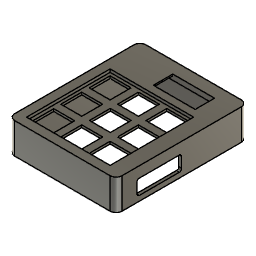
bdn9-top-case (Autodesk Fusion 360 design; units mm, degrees)
Autodesk Fusion 360 part; units mm, degrees
note: some values were not read from the file. Chosen so that the rebuilt part matches the saved one: which face or edge a step refers to; which pieces of a blend or face edit are solid.
sketch "Sketch1" plane through (0, 0, 0) normal (0, 0, 1) x (1, 0, 0)
  line L0 (-8, -80) -> (-22, -80)
  line L1 (-22, -80) -> (-22, -66)
  line L2 (-22, -66) -> (-8, -66)
  line L3 (-8, -66) -> (-8, -80)
  line L4 (-8, -61) -> (-22, -61)
  line L5 (-22, -61) -> (-22, -47)
  line L6 (-22, -47) -> (-8, -47)
  line L7 (-8, -47) -> (-8, -61)
  line L8 (-8, -42) -> (-22, -42)
  line L9 (-22, -42) -> (-22, -28)
  line L10 (-22, -28) -> (-8, -28)
  line L11 (-8, -28) -> (-8, -42)
  line L12 (0, 0) -> (-68, 0)
  line L13 (-68, 0) -> (-68, -88)
  line L14 (-68, -88) -> (0, -88)
  line L15 (0, -88) -> (0, 0)
  line L16 (-27, -28) -> (-41, -28)
  line L17 (-41, -28) -> (-41, -42)
  line L18 (-41, -42) -> (-27, -42)
  line L19 (-27, -42) -> (-27, -28)
  line L20 (-27, -46.8468) -> (-41, -46.8468)
  line L21 (-41, -46.8468) -> (-41, -60.8468)
  line L22 (-41, -60.8468) -> (-27, -60.8468)
  line L23 (-27, -60.8468) -> (-27, -46.8468)
  line L24 (-27, -66) -> (-41, -66)
  line L25 (-41, -66) -> (-41, -80)
  line L26 (-41, -80) -> (-27, -80)
  line L27 (-27, -80) -> (-27, -66)
  line L28 (-46, -28) -> (-60, -28)
  line L29 (-60, -28) -> (-60, -42)
  line L30 (-60, -42) -> (-46, -42)
  line L31 (-46, -42) -> (-46, -28)
  line L32 (-46, -47) -> (-60, -47)
  line L33 (-60, -47) -> (-60, -61)
  line L34 (-60, -61) -> (-46, -61)
  line L35 (-46, -61) -> (-46, -47)
  line L36 (-45.7846, -66) -> (-59.7846, -66)
  line L37 (-59.7846, -66) -> (-59.7846, -80)
  line L38 (-59.7846, -80) -> (-45.7846, -80)
  line L39 (-45.7846, -80) -> (-45.7846, -66)
  line L40 (-5, -8) -> (-44, -8)
  line L41 (-44, -8) -> (-44, -21)
  line L42 (-44, -21) -> (-5, -21)
  line L43 (-5, -21) -> (-5, -8)
  dimension "d15" = 68
  dimension "d16" = 88
  dimension "d29" = 39
  dimension "d30" = 13
  constraint horizontal L0
  constraint vertical L1
  constraint horizontal L2
  constraint vertical L3
  constraint horizontal L4
  constraint vertical L5
  constraint horizontal L6
  constraint vertical L7
  constraint horizontal L8
  constraint vertical L9
  constraint horizontal L10
  constraint vertical L11
  constraint horizontal L12
  constraint vertical L13
  constraint horizontal L14
  constraint vertical L15
  constraint coincident L12.start L15.end
  constraint horizontal L16
  constraint vertical L17
  constraint horizontal L18
  constraint vertical L19
  constraint horizontal L20
  constraint vertical L21
  constraint horizontal L22
  constraint vertical L23
  constraint horizontal L24
  constraint vertical L25
  constraint horizontal L26
  constraint vertical L27
  constraint horizontal L28
  constraint vertical L29
  constraint horizontal L30
  constraint vertical L31
  constraint horizontal L32
  constraint vertical L33
  constraint horizontal L34
  constraint vertical L35
  constraint horizontal L36
  constraint vertical L37
  constraint horizontal L38
  constraint vertical L39
  constraint horizontal L40
  constraint vertical L41
  constraint horizontal L42
  constraint vertical L43
  measures "d15" distance of L12.start L12.end
  measures "d16" distance of L12.start L14.end
  measures "d29" distance of L40.start L40.end
  measures "d30" distance of L40.start L42.end
extrude "Extrude1" add sketch "Sketch1" along normal blind 2
extrude "Extrude2" cut 1 faces at (-57.3333, -12, 2) along direction (0, 0, -1) blind 0.4
extrude "Extrude3" add 1 faces at (0, -58.6667, 0.5333) along direction (1, 0, 0) blind 2
sketch "Sketch2" plane through (0, 0, 1.6) normal (0, 0, 1) x (-1, 0, 0)
  line L0 (27, 66) -> (27, 80)
  line L1 (27, 80) -> (41, 80)
  line L2 (41, 80) -> (41, 66)
  line L3 (41, 66) -> (27, 66)
  line L4 (5, 8) -> (5, 21)
  line L5 (5, 21) -> (44, 21)
  line L6 (44, 21) -> (44, 8)
  line L7 (44, 8) -> (5, 8)
  line L8 (27, 46.8468) -> (27, 60.8468)
  line L9 (27, 60.8468) -> (41, 60.8468)
  line L10 (41, 60.8468) -> (41, 46.8468)
  line L11 (41, 46.8468) -> (27, 46.8468)
  line L12 (22, 47) -> (8, 47)
  line L13 (8, 47) -> (8, 61)
  line L14 (8, 61) -> (22, 61)
  line L15 (22, 61) -> (22, 47)
  line L16 (22, 66) -> (8, 66)
  line L17 (8, 66) -> (8, 80)
  line L18 (8, 80) -> (22, 80)
  line L19 (22, 80) -> (22, 66)
  line L20 (27, 28) -> (27, 42)
  line L21 (27, 42) -> (41, 42)
  line L22 (41, 42) -> (41, 28)
  line L23 (41, 28) -> (27, 28)
  line L24 (22, 28) -> (8, 28)
  line L25 (8, 28) -> (8, 42)
  line L26 (8, 42) -> (22, 42)
  line L27 (22, 42) -> (22, 28)
  line L28 (46, 47) -> (46, 61)
  line L29 (46, 61) -> (60, 61)
  line L30 (60, 61) -> (60, 47)
  line L31 (60, 47) -> (46, 47)
  line L32 (46, 28) -> (46, 42)
  line L33 (46, 42) -> (60, 42)
  line L34 (60, 42) -> (60, 28)
  line L35 (60, 28) -> (46, 28)
  line L36 (45.7846, 66) -> (45.7846, 80)
  line L37 (45.7846, 80) -> (59.7846, 80)
  line L38 (59.7846, 80) -> (59.7846, 66)
  line L39 (59.7846, 66) -> (45.7846, 66)
  line L40 (-2, 0) -> (68, 0)
  line L41 (68, 0) -> (68, 88)
  line L42 (68, 88) -> (-2, 88)
  line L43 (-2, 88) -> (-2, 0)
  line L44 (6, 26) -> (62, 26)
  line L45 (62, 26) -> (62, 82)
  line L46 (62, 82) -> (6, 82)
  line L47 (6, 82) -> (6, 26)
  constraint horizontal L44
  constraint vertical L45
  constraint horizontal L46
  constraint vertical L47
extrude "Extrude4" add sketch "Sketch2" along normal blind 2 contours L40 L41 L42 L43
sketch "Sketch3" plane through (0, 0, 0) normal (0, 0, 1) x (1, 0, 0)
  line L0 (-10, -8) -> (-38, -8)
  line L1 (-38, -8) -> (-38, -21)
  line L2 (-38, -21) -> (-10, -21)
  line L3 (-10, -21) -> (-10, -8)
  line L4 (-38, -8) -> (-44, -8)
  line L5 (-44, -8) -> (-44, -21)
  line L6 (-44, -21) -> (-38, -21)
  line L7 (-38, -21) -> (-38, -8)
  line L8 (-10, -8) -> (-5, -8)
  line L9 (-5, -8) -> (-5, -21)
  line L10 (-5, -21) -> (-10, -21)
  line L11 (-10, -21) -> (-10, -8)
  dimension "d39" = 28
  dimension "d40" = 13
  constraint horizontal L0
  constraint vertical L1
  constraint horizontal L2
  constraint vertical L3
  constraint horizontal L4
  constraint vertical L5
  constraint horizontal L6
  constraint vertical L7
  constraint horizontal L8
  constraint vertical L9
  constraint horizontal L10
  constraint vertical L11
  measures "d39" distance of L0.start L0.end
  measures "d40" distance of L0.start L2.end
move_body "Move1" bodies 1 to x (1, 0, 0) y (0, 1, 0) z (0, 0, 1) at (0, 0, -3)
extrude "Extrude5" add sketch "Sketch3" along normal blind 0.6 contours L3 L8 L9 L10 L11 | L1 L4 L5 L6 L7
extrude "Extrude6" add 2 faces at (-42, -16.6667, 0) (-6.6667, -16.6667, 0) along direction (0, 0, -1) blind 0.4
sketch "Sketch4" plane through (0, 0, 0) normal (0, 0, 1) x (1, 0, 0)
move_body "Move2" bodies 1 to x (1, 0, 0) y (0, 1, 0) z (0, 0, 1) at (0, 0, 0.6)
sketch "Sketch5" plane through (0, 0, 0) normal (0, 0, 1) x (1, 0, 0)
sketch "Sketch6" plane through (0, 0, 0) normal (0, 0, 1) x (1, 0, 0)
sketch "Sketch7" plane through (0, 0, -2.4) normal (0, 0, -1) x (1, 0, 0)
  line L0 (-27, 80) -> (-27, 66)
  line L1 (-27, 66) -> (-41, 66)
  line L2 (-41, 66) -> (-41, 80)
  line L3 (-41, 80) -> (-27, 80)
  line L4 (-5, 21) -> (-5, 8)
  line L5 (-5, 8) -> (-44, 8)
  line L6 (-44, 8) -> (-44, 21)
  line L7 (-44, 21) -> (-5, 21)
  line L8 (-27, 60.8468) -> (-27, 46.8468)
  line L9 (-27, 46.8468) -> (-41, 46.8468)
  line L10 (-41, 46.8468) -> (-41, 60.8468)
  line L11 (-41, 60.8468) -> (-27, 60.8468)
  line L12 (-8, 47) -> (-22, 47)
  line L13 (-22, 47) -> (-22, 61)
  line L14 (-22, 61) -> (-8, 61)
  line L15 (-8, 61) -> (-8, 47)
  line L16 (-8, 66) -> (-22, 66)
  line L17 (-22, 66) -> (-22, 80)
  line L18 (-22, 80) -> (-8, 80)
  line L19 (-8, 80) -> (-8, 66)
  line L20 (-27, 42) -> (-27, 28)
  line L21 (-27, 28) -> (-41, 28)
  line L22 (-41, 28) -> (-41, 42)
  line L23 (-41, 42) -> (-27, 42)
  line L24 (-8, 28) -> (-22, 28)
  line L25 (-22, 28) -> (-22, 42)
  line L26 (-22, 42) -> (-8, 42)
  line L27 (-8, 42) -> (-8, 28)
  line L28 (-46, 61) -> (-46, 47)
  line L29 (-46, 47) -> (-60, 47)
  line L30 (-60, 47) -> (-60, 61)
  line L31 (-60, 61) -> (-46, 61)
  line L32 (-46, 42) -> (-46, 28)
  line L33 (-46, 28) -> (-60, 28)
  line L34 (-60, 28) -> (-60, 42)
  line L35 (-60, 42) -> (-46, 42)
  line L36 (-45.7846, 80) -> (-45.7846, 66)
  line L37 (-45.7846, 66) -> (-59.7846, 66)
  line L38 (-59.7846, 66) -> (-59.7846, 80)
  line L39 (-59.7846, 80) -> (-45.7846, 80)
  line L40 (2, 88) -> (-68, 88)
  line L41 (-68, 88) -> (-68, 0)
  line L42 (-68, 0) -> (2, 0)
  line L43 (2, 0) -> (2, 88)
sketch "Sketch8" plane through (0, 0, 0) normal (0, 0, 1) x (1, 0, 0)
sketch "Sketch9" plane through (0, 0, -2.4) normal (0, 0, -1) x (1, 0, 0)
  line L0 (-2, 84) -> (-64, 84)
  line L1 (-64, 84) -> (-64, 4)
  line L2 (-64, 4) -> (-2, 4)
  line L3 (-2, 4) -> (-2, 84)
  constraint horizontal L0
  constraint vertical L1
  constraint horizontal L2
  constraint vertical L3
extrude "Extrude7" add sketch "Sketch7" along normal blind 17
extrude "Extrude8" cut sketch "Sketch9" along normal blind 17
sketch "Sketch10" plane through (2, 0, 0) normal (1, 0, 0) x (0, 1, 0)
  line L0 (-88, 1.2) -> (-88, -19.4)
  line L1 (-88, -19.4) -> (0, -19.4)
  line L2 (0, -19.4) -> (0, 1.2)
  line L3 (0, 1.2) -> (-88, 1.2)
sketch "Sketch11" plane through (2, 0, 0) normal (1, 0, 0) x (0, 1, 0)
  line L0 (-68, -16) -> (-38, -16)
  line L1 (-38, -16) -> (-38, -6)
  line L2 (-38, -6) -> (-68, -6)
  line L3 (-68, -6) -> (-68, -16)
  dimension "d49" = 30
  dimension "d50" = 10
  constraint horizontal L0
  constraint vertical L1
  constraint horizontal L2
  constraint vertical L3
  measures "d49" distance of L0.start L0.end
  measures "d50" distance of L0.start L2.end
extrude "Extrude9" cut sketch "Sketch11" against normal blind 4
fillet "Fillet1" radius 1.5 1 edges at (0, -68, -6)
fillet "Fillet2" radius 1.5 1 edges at (0, -38, -6)
fillet "Fillet3" radius 1.5 1 edges at (0, -68, -16)
fillet "Fillet4" radius 1.5 1 edges at (0, -38, -16)
fillet "Fillet5" radius 4 1 edges at (2, -88, -9.1)
fillet "Fillet6" radius 4 1 edges at (2, 0, -9.1)
fillet "Fillet7" radius 4 1 edges at (-68, 0, -9.1)
fillet "Fillet8" radius 4 1 edges at (-68, -88, -9.1)
sketch "Sketch12" plane through (0, 0, 0) normal (0, 0, 1) x (1, 0, 0)
  line L0 (-2, -4, -19.4) -> (-11, -4, -19.4)
  line L1 (-11, -4, -19.4) -> (-11, -13, -19.4)
  line L2 (-11, -13, -19.4) -> (-2, -13, -19.4)
  line L3 (-2, -13, -19.4) -> (-2, -4, -19.4)
  dimension "d61" = 9
  dimension "d62" = 9
sketch "Sketch13" plane through (0, 0, -19.4) normal (0, 0, 1) x (1, 0, 0)
  line L0 (-64, -4) -> (-55, -4)
  line L1 (-55, -4) -> (-55, -13)
  line L2 (-55, -13) -> (-64, -13)
  line L3 (-64, -13) -> (-64, -4)
  line L4 (-64, -84) -> (-55, -84)
  line L5 (-55, -84) -> (-55, -75)
  line L6 (-55, -75) -> (-64, -75)
  line L7 (-64, -75) -> (-64, -84)
  line L8 (-2, -84) -> (-11, -84)
  line L9 (-11, -84) -> (-11, -75)
  line L10 (-11, -75) -> (-2, -75)
  line L11 (-2, -75) -> (-2, -84)
  point P0 (-64, -4)
  point P1 (-64, -84)
  point P2 (-2, -84)
  dimension "d63" = 9
  dimension "d64" = 9
  dimension "d65" = 9
  dimension "d66" = 9
  dimension "d67" = 9
  dimension "d68" = 9
  constraint horizontal L0
  constraint vertical L1
  constraint horizontal L2
  constraint vertical L3
  constraint coincident P0 L0.start
  constraint horizontal L4
  constraint vertical L5
  constraint horizontal L6
  constraint vertical L7
  constraint coincident P1 L4.start
  constraint horizontal L8
  constraint vertical L9
  constraint horizontal L10
  constraint vertical L11
  constraint coincident P2 L8.start
  measures "d63" distance of P0 L0.end
  measures "d64" distance of P0 L2.end
  measures "d65" distance of P1 L4.end
  measures "d66" distance of P1 L6.end
  measures "d67" distance of P2 L8.end
  measures "d68" distance of P2 L10.end
sketch "Sketch12 (curves -19.4 mm off its plane)" plane through (0, 0, -19.4) normal (0, 0, 1) x (1, 0, 0)
  line L0 (-2, -4) -> (-11, -4)
  line L1 (-11, -4) -> (-11, -13)
  line L2 (-11, -13) -> (-2, -13)
  line L3 (-2, -13) -> (-2, -4)
extrude "Extrude10" add sketch "Sketch12 (curves -19.4 mm off its plane)" along normal blind 1
move_face "MoveFace1" by (0, 0, 1) 3 faces at (-11, -7, -19.0667) (-8, -13, -19.0667) (-8, -7, -18.4)
sketch "Sketch14" plane through (0, 0, -19.4) normal (0, 0, -1) x (1, 0, 0)
  line L0 (-11, 4) -> (-64, 4)
  line L1 (-64, 4) -> (-64, 84)
  line L2 (-64, 84) -> (-2, 84)
  line L3 (-2, 84) -> (-2, 13)
  line L4 (-2, 13) -> (-11, 13)
  line L5 (-11, 13) -> (-11, 4)
  arc A0 (-64, 88) -> (-68, 84) centre (-64, 84) ccw
  line L6 (-68, 84) -> (-68, 4)
  arc A1 (-68, 4) -> (-64, 0) centre (-64, 4) ccw
  line L7 (-64, 0) -> (-2, 0)
  arc A2 (-2, 0) -> (2, 4) centre (-2, 4) ccw
  line L8 (2, 4) -> (2, 84)
  arc A3 (2, 84) -> (-2, 88) centre (-2, 84) ccw
  line L9 (-2, 88) -> (-64, 88)
  line L10 (-11, 4) -> (-2, 4)
  line L11 (-2, 4) -> (-2, 13)
  line L12 (-2, 13) -> (-11, 13)
  line L13 (-11, 13) -> (-11, 4)
  constraint horizontal L10
  constraint vertical L11
  constraint horizontal L12
  constraint vertical L13
  constraint coincident L3.end L4.start
  constraint coincident L0.start L5.end
extrude "Extrude11" cut sketch "Sketch14" against normal blind 1 contours L4 L5 L10 L11 L12 L13
extrude "Extrude12" add sketch "Sketch13" along normal blind 2 contours L0 L1 L2 L3
sketch "Sketch15" plane through (0, 0, -19.4) normal (0, 0, -1) x (1, 0, 0)
  line L0 (-2, 4) -> (-55, 4)
  line L1 (-55, 4) -> (-55, 13)
  line L2 (-55, 13) -> (-64, 13)
  line L3 (-64, 13) -> (-64, 84)
  line L4 (-64, 84) -> (-2, 84)
  line L5 (-2, 84) -> (-2, 4)
  arc A0 (-64, 88) -> (-68, 84) centre (-64, 84) ccw
  line L6 (-68, 84) -> (-68, 4)
  arc A1 (-68, 4) -> (-64, 0) centre (-64, 4) ccw
  line L7 (-64, 0) -> (-2, 0)
  arc A2 (-2, 0) -> (2, 4) centre (-2, 4) ccw
  line L8 (2, 4) -> (2, 84)
  arc A3 (2, 84) -> (-2, 88) centre (-2, 84) ccw
  line L9 (-2, 88) -> (-64, 88)
  line L10 (-64, 13) -> (-55, 13)
  line L11 (-55, 13) -> (-55, 4)
  line L12 (-55, 4) -> (-64, 4)
  line L13 (-64, 4) -> (-64, 13)
  constraint horizontal L10
  constraint vertical L11
  constraint horizontal L12
  constraint vertical L13
  constraint coincident L0.end L1.start
  constraint coincident L2.end L3.start
extrude "Extrude13" cut sketch "Sketch15" against normal blind 1 contours L1 L2 L10 L11 L12 L13
extrude "Extrude14" add 1 faces at (-61, -7, -17.4) along direction (0, 0, 1) blind 2.5
extrude "Extrude15" cut 1 faces at (-58, -7, -18.4) along direction (0, 0, 1) blind 1
sketch "Sketch16" plane through (0, 0, -19.4) normal (0, 0, -1) x (1, 0, 0)
  line L0 (-64, 4) -> (-64, 84)
  line L1 (-64, 84) -> (-2, 84)
  line L2 (-2, 84) -> (-2, 4)
  line L3 (-2, 4) -> (-64, 4)
  arc A0 (-64, 88) -> (-68, 84) centre (-64, 84) ccw
  line L4 (-68, 84) -> (-68, 4)
  arc A1 (-68, 4) -> (-64, 0) centre (-64, 4) ccw
  line L5 (-64, 0) -> (-2, 0)
  arc A2 (-2, 0) -> (2, 4) centre (-2, 4) ccw
  line L6 (2, 4) -> (2, 84)
  arc A3 (2, 84) -> (-2, 88) centre (-2, 84) ccw
  line L7 (-2, 88) -> (-64, 88)
  line L8 (-64, 84) -> (-55, 84)
  line L9 (-55, 84) -> (-55, 75)
  line L10 (-55, 75) -> (-64, 75)
  line L11 (-64, 75) -> (-64, 84)
  dimension "d81" = 9
  dimension "d82" = 9
  constraint horizontal L8
  constraint vertical L9
  constraint horizontal L10
  constraint vertical L11
  constraint coincident L0.end L1.start
  measures "d81" distance of L0.end L8.end
  measures "d82" distance of L0.end L10.end
extrude "Extrude16" add sketch "Sketch16" against normal blind 4.5 contours L0 L1 L8 L9 L10 L11
sketch "Sketch17" plane through (0, 0, -19.4) normal (0, 0, -1) x (1, 0, 0)
  line L0 (-64, 4) -> (-64, 75)
  line L1 (-64, 75) -> (-55, 75)
  line L2 (-55, 75) -> (-55, 84)
  line L3 (-55, 84) -> (-2, 84)
  line L4 (-2, 84) -> (-2, 4)
  line L5 (-2, 4) -> (-64, 4)
  arc A0 (-64, 88) -> (-68, 84) centre (-64, 84) ccw
  line L6 (-68, 84) -> (-68, 4)
  arc A1 (-68, 4) -> (-64, 0) centre (-64, 4) ccw
  line L7 (-64, 0) -> (-2, 0)
  arc A2 (-2, 0) -> (2, 4) centre (-2, 4) ccw
  line L8 (2, 4) -> (2, 84)
  arc A3 (2, 84) -> (-2, 88) centre (-2, 84) ccw
  line L9 (-2, 88) -> (-64, 88)
  line L10 (-55, 84) -> (-64, 84)
  line L11 (-64, 84) -> (-64, 75)
  line L12 (-64, 75) -> (-55, 75)
  line L13 (-55, 75) -> (-55, 84)
  constraint horizontal L10
  constraint vertical L11
  constraint horizontal L12
  constraint vertical L13
  constraint coincident L0.end L1.start
  constraint coincident L2.end L3.start
extrude "Extrude17" cut sketch "Sketch17" against normal blind 2 contours L1 L2 L10 L11 L12 L13
sketch "Sketch18" plane through (0, 0, -19.4) normal (0, 0, -1) x (1, 0, 0)
  arc A0 (-64, 88) -> (-68, 84) centre (-64, 84) ccw
  line L0 (-68, 84) -> (-68, 4)
  arc A1 (-68, 4) -> (-64, 0) centre (-64, 4) ccw
  line L1 (-64, 0) -> (-2, 0)
  arc A2 (-2, 0) -> (2, 4) centre (-2, 4) ccw
  line L2 (2, 4) -> (2, 84)
  arc A3 (2, 84) -> (-2, 88) centre (-2, 84) ccw
  line L3 (-2, 88) -> (-64, 88)
  line L4 (-64, 4) -> (-64, 84)
  line L5 (-64, 84) -> (-2, 84)
  line L6 (-2, 84) -> (-2, 4)
  line L7 (-2, 4) -> (-64, 4)
  line L8 (-2, 84) -> (-11, 84)
  line L9 (-11, 84) -> (-11, 75)
  line L10 (-11, 75) -> (-2, 75)
  line L11 (-2, 75) -> (-2, 84)
  dimension "d87" = 9
  dimension "d88" = 9
  constraint horizontal L8
  constraint vertical L9
  constraint horizontal L10
  constraint vertical L11
  constraint coincident A3.centre L5.end
  measures "d87" distance of A3.centre L8.end
  measures "d88" distance of A3.centre L10.end
extrude "Extrude18" add sketch "Sketch18" against normal blind 4.5 contours L5 L6 L8 L9 L10 L11
sketch "Sketch19" plane through (0, 0, -19.4) normal (0, 0, -1) x (1, 0, 0)
  arc A0 (-64, 88) -> (-68, 84) centre (-64, 84) ccw
  line L0 (-68, 84) -> (-68, 4)
  arc A1 (-68, 4) -> (-64, 0) centre (-64, 4) ccw
  line L1 (-64, 0) -> (-2, 0)
  arc A2 (-2, 0) -> (2, 4) centre (-2, 4) ccw
  line L2 (2, 4) -> (2, 84)
  arc A3 (2, 84) -> (-2, 88) centre (-2, 84) ccw
  line L3 (-2, 88) -> (-64, 88)
  line L4 (-64, 4) -> (-64, 84)
  line L5 (-64, 84) -> (-11, 84)
  line L6 (-11, 84) -> (-11, 75)
  line L7 (-11, 75) -> (-2, 75)
  line L8 (-2, 75) -> (-2, 4)
  line L9 (-2, 4) -> (-64, 4)
  line L10 (-2, 75) -> (-11, 75)
  line L11 (-11, 75) -> (-11, 84)
  line L12 (-11, 84) -> (-2, 84)
  line L13 (-2, 84) -> (-2, 75)
  constraint horizontal L10
  constraint vertical L11
  constraint horizontal L12
  constraint vertical L13
  constraint coincident L5.end L6.start
  constraint coincident L7.end L8.start
extrude "Extrude19" cut sketch "Sketch19" against normal blind 2 contours L6 L7 L10 L11 L12 L13
extrude "Extrude20" add 1 faces at (-8, -7, -17.4) along direction (0, 0, 1) blind 2.5
extrude "Extrude21" cut 1 faces at (-8, -7, -18.4) along direction (0, 0, 1) blind 1
delete_face "DeleteFace1" 1 faces at (-1.6198, -0.0181, -5.6667)
delete_face "DeleteFace2" 1 faces at (1.9819, -84.3802, -12.5333)
extrude "Extrude22" add sketch "Sketch10" along normal blind 2
extrude "Extrude23" cut 1 faces at (2, -48.5, -12.6667) along direction (1, 0, 0) blind 2
extrude "Extrude24" cut 1 faces at (-2, -18.3785, -8.059) along direction (1, 0, 0) blind 2
extrude "Extrude25" cut 1 faces at (0, -18.3785, -8.059) along direction (1, 0, 0) blind 2
fillet "Fillet9" radius 4 1 edges at (4, -88, -9.1)
fillet "Fillet10" radius 4 1 edges at (4, 0, -9.1)
move_face "MoveFace2" to x (1, 0, 0) y (0, 1, 0) z (0, 0, 1) at (0, -6, 0) 6 faces at (2.6667, -38, -12.1667) (3.3333, -38.4649, -6.4144) (3.3333, -67.3701, -6.2781) (3.3333, -68, -9.8333) (3.3333, -67.4272, -15.6791) (3.3333, -39.4286, -15.9983)
